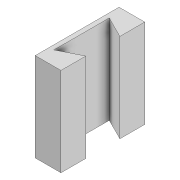
# Autodesk Inventor part: Sliding test receiver
Saved by Autodesk Inventor 2020 (Build 240168000, 168)
## iProperties
Created: 2019-11-10
Part Number: Sliding test receiver
Material: Generic
Document SubType Name: Modeling
Designer: ball
Density: 1 g/cm^3
Appearance: Default
Author: ball
Autodesk Inventor part; units mm, degrees
ref_plane "YZ Plane" through (0, 0, 0) normal (1, 0, 0) x (0, 1, 0)
ref_plane "XZ Plane" through (0, 0, 0) normal (0, 1, 0) x (-1, 0, 0)
ref_plane "XY Plane" through (0, 0, 0) normal (0, 0, 1) x (1, 0, 0)
sketch "Sketch1" plane through (0, 0, 0) normal (0, 1, 0) x (-1, 0, 0)
  line L0 (0, 12) -> (7.366, 12)
  line L1 (7.366, 12) -> (7.366, -12)
  line L2 (7.366, -12) -> (0, -12)
  line L3 (6.096, 4.881) -> (6.096, -4.881)
  line L4 (0, 4.881) -> (0, 7.929)
  line L5 (6.096, 7.929) -> (6.096, 4.881)
  line L6 (0, -4.881) -> (0, -7.548)
  line L7 (6.096, -7.929) -> (6.096, -4.881)
  line L8 (6.096, 7.929) -> (0, 4.881)
  line L9 (6.096, -7.929) -> (0, -4.881)
  line L10 (0, -12) -> (0, -4.881)
  line L11 (0, 4.881) -> (0, 12)
  point P0 (0, 0)
  dimension "d0" = 7.366
  dimension "d1" = 24
  dimension "d2" = 12
  dimension "d8" = 9.762
  dimension "d9" = 4.881
  dimension "d10" = 3.048
  dimension "d11" = 3.048
  dimension "d12" = 6.096
  constraints: 24 end point, 5 parallel, 2 point on line, 1 horizontal, 1 perpendicular
  measures "d0" distance of L1.end L2.end
  measures "d1" distance of L0.end L1.end
  measures "d2" distance from line of L0 point (0, 0)
  measures "d8" distance of L6.start L4.start
  measures "d9" distance of point (0, 0) L4.start
  measures "d10" vertical distance of L5.start L4.start
  measures "d11" vertical distance of L7.start L6.start
  measures "d12" distance from line of L10 L7.start
extrude "Extrusion1" add sketch "Sketch1" along normal blind 25.4
equation "\"d2\" = 0.5 * d1"
equation "\"d9\" = 0.5 * d8"
equation "\"d11\" = d10"
body "Solid1"
